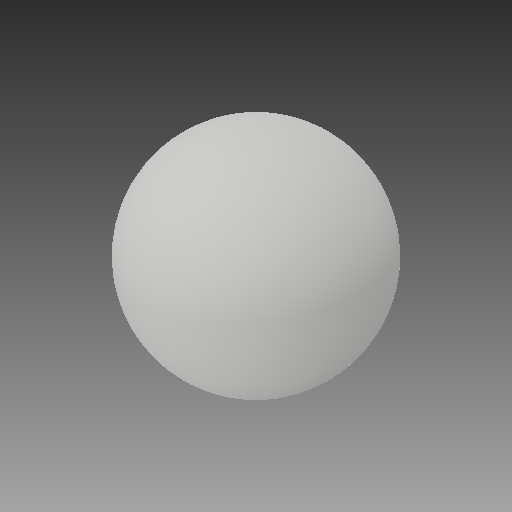
# Autodesk Inventor part: Food-Grade Abrasion-Resistant Natural Rubber Ball 5-8 in
Saved by Autodesk Inventor 2018 (Build 220112000, 112)
## iProperties
Created: 2020-03-28
Part Number: Food-Grade Abrasion-Resistant Natural Rubber Ball 5-8 in
Material: Generic
Document SubType Name: Modeling
Designer: emile
Density: 1 g/cm^3
Appearance: Default
Catalog Web Link: https://www.mcmaster.com/96385k61
Mass: 2.09479 g
Surface Area: 7.9173 cm^2
Volume: 2.09479 cm^3
Author: emile
Autodesk Inventor part; units mm, degrees
ref_plane "YZ Plane" through (0, 0, 0) normal (1, 0, 0) x (0, 1, 0)
ref_plane "XZ Plane" through (0, 0, 0) normal (0, 1, 0) x (-1, 0, 0)
ref_plane "XY Plane" through (0, 0, 0) normal (0, 0, 1) x (1, 0, 0)
sketch "Sketch1" plane through (0, 0, 0) normal (1, 0, 0) x (0, 1, 0)
  circle A0 centre (0, 0) radius 7.9375
  line L0 (0, 7.9375) -> (0, -7.9375)
  dimension "d0" = 15.875
  constraints: 2 end point, 2 point on circle, 1 centre point, 1 coincident, 1 midpoint, 1 vertical
  measures "d0" diameter of A0
revolve "Revolution1" add sketch "Sketch1" angle 360 about axis through (0, 0, 7.9375) along (0, 0, -1) picked at (2.0686, 1.6497) contours A0 L0
body "Solid1"
